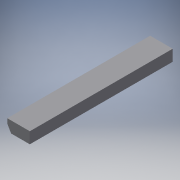
# Autodesk Inventor part: front_screen_footer
Saved by Autodesk Inventor 2017 (Build 210142000, 142)
## iProperties
Created: 2019-03-22
Part Number: front_screen_footer
Material: Generic
Document SubType Name: Modeling
Designer: Mitch
Density: 1 g/cm^3
Appearance: Default
Author: Mitch
Autodesk Inventor part; units mm, degrees
ref_plane "YZ Plane" through (0, 0, 0) normal (1, 0, 0) x (0, 1, 0)
ref_plane "XZ Plane" through (0, 0, 0) normal (0, 1, 0) x (-1, 0, 0)
ref_plane "XY Plane" through (0, 0, 0) normal (0, 0, 1) x (1, 0, 0)
sketch "Sketch1" plane through (0, 0, 0) normal (0, 1, 0) x (-1, 0, 0)
  line L0 (0, 0) -> (38.1, 0)
  line L1 (38.1, 0) -> (38.1, -241.3)
  line L2 (38.1, -241.3) -> (0, -241.3)
  line L3 (0, -241.3) -> (0, 0)
  dimension "d0" = 38.1
  dimension "d1" = 241.3
  constraints: 8 end point, 2 parallel, 1 horizontal, 1 perpendicular
  measures "d0" distance of L1.end L2.end
  measures "d1" distance of L0.end L1.end
extrude "Extrusion1" add sketch "Sketch1" along normal blind 19.05
sketch "Sketch2" plane through (0, 0, -241.3) normal (0, 0, -1) x (-1, 0, 0)
  line L0 (204.3257, -100.8201) -> (38.1, 11.3005) projected
  line L1 (38.1, 11.3005) -> (31.5757, 0)
  line L2 (0, 0) -> (38.1, 0) projected
  line L3 (38.1, 11.3005) -> (51.1487, 11.3005) construction
  line L4 (31.5757, 0) -> (38.1, 0)
  line L5 (38.1, 0) -> (38.1, 11.3005)
  dimension "d4" = 120
  constraints: 8 end point, 1 collinear, 1 equal length, 1 horizontal, 1 perpendicular, 1 point on line
  measures "d4" angle of L1 L3
extrude "Extrusion2" cut sketch "Sketch2" against normal blind 241.3
body "Solid1"
